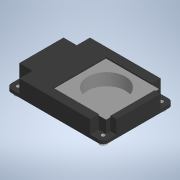
# Autodesk Inventor part: PRI_cooler
Saved by Autodesk Inventor 2022 (Build 260153000, 153)
## iProperties
Created: 2025-03-29
Part Number: PRI_cooler
Material: Типовые
Document SubType Name: Modeling
Designer: akap
Density: 1 g/cm^3
Appearance: По умолчанию
Author: akap
Autodesk Inventor part; units mm, degrees
ref_plane "YZ Plane" through (0, 0, 0) normal (1, 0, 0) x (0, 1, 0)
ref_plane "XZ Plane" through (0, 0, 0) normal (0, 1, 0) x (-1, 0, 0)
ref_plane "XY Plane" through (0, 0, 0) normal (0, 0, 1) x (1, 0, 0)
sketch "Эскиз1" plane through (0, 0, 0) normal (0, 1, 0) x (-1, 0, 0)
  line L0 (-24.5, 20) -> (24.5, 20)
  line L1 (27.5, 17) -> (27.5, -17)
  line L2 (24.5, -20) -> (-24.5, -20)
  line L3 (-27.5, -17) -> (-27.5, 17)
  line L4 (-27.5, 20) -> (27.5, -20) construction
  line L5 (27.5, 20) -> (-27.5, -20) construction
  arc A0 (24.5, -20) -> (27.5, -17) centre (24.5, -17) ccw
  arc A1 (-27.5, -17) -> (-24.5, -20) centre (-24.5, -17) ccw
  arc A2 (-24.5, 20) -> (-27.5, 17) centre (-24.5, 17) ccw
  arc A3 (27.5, 17) -> (24.5, 20) centre (24.5, 17) ccw
  line L6 (-24, 16.5) -> (24, 16.5)
  line L7 (24, 16.5) -> (24, -16.5)
  line L8 (24, -16.5) -> (-24, -16.5)
  line L9 (-24, -16.5) -> (-24, 16.5)
  line L10 (-24, 16.5) -> (24, -16.5) construction
  line L11 (24, 16.5) -> (-24, -16.5) construction
  circle A4 centre (24, 16.5) radius 1
  circle A5 centre (24, -16.5) radius 1
  circle A6 centre (-24, -16.5) radius 1
  circle A7 centre (-24, 16.5) radius 1
  point P0 (0, 0)
  dimension "d0" = 55
  dimension "d1" = 40
  dimension "d2" = 3
  dimension "d3" = 3
  dimension "d30" = 48
  dimension "d31" = 33
  dimension "d32" = 2
  dimension "d33" = 2
  dimension "d34" = 2
  dimension "d35" = 2
  constraints: 24 end point, 8 centre point, 8 point on circle, 8 point on line, 8 tangent, 4 coincident, 4 midpoint, 4 parallel, 2 equal radius, 2 horizontal, 2 perpendicular
  measures "d0" distance of L4.end L5.end
  measures "d1" distance of L5.start L4.end
  measures "d2" radius of A0
  measures "d3" radius of A3
  measures "d30" distance of L7.end L8.end
  measures "d31" distance of L6.end L7.end
  measures "d32" diameter of A4
  measures "d33" diameter of A5
  measures "d34" diameter of A6
  measures "d35" diameter of A7
extrude "Выдавливание1" add sketch "Эскиз1" along normal blind 1.8 contours L0 A3 L1 A0 L2 A1 L3 A2 | L6 A4 L7 A5 L8 A6 L9 A7
sketch "Эскиз2" plane through (0, 1.8, 0) normal (0, 1, 0) x (1, 0, 0)
  line L0 (-5.9, 15) -> (24.1, 15)
  line L1 (24.1, 15) -> (24.1, -15)
  line L2 (24.1, -15) -> (-5.9, -15)
  line L3 (-5.9, -15) -> (-5.9, 15)
  line L4 (-5.9, 15) -> (24.1, -15) construction
  line L5 (24.1, 15) -> (-5.9, -15) construction
  line L6 (27.5, -17) -> (27.5, 17) projected
  line L7 (-27.5, 17) -> (-27.5, -17) projected
  line L8 (-27.5, 0) -> (27.5, 0)
  circle A0 centre (8.45, 0.95) radius 10.65
  line L9 (8.45, 15) -> (8.45, 0.95)
  line L10 (8.45, 11.6) -> (8.45, 15)
  line L11 (-5.9, 0.95) -> (8.45, 0.95)
  line L12 (-5.9, 0.95) -> (-2.2, 0.95)
  point P0 (0, 0)
  point P1 (9.1, 0)
  dimension "d10" = 30
  dimension "d11" = 30
  dimension "d12" = 3.4
  dimension "d13" = 21.3
  dimension "d14" = 3.4
  dimension "d15" = 3.7
  constraints: 22 end point, 7 point on line, 4 midpoint, 2 horizontal, 2 parallel, 2 perpendicular, 2 point on circle, 1 centre point
  measures "d10" distance of L1.end L2.end
  measures "d11" distance of L0.end L1.end
  measures "d12" distance between parallel lines of L6 L1
  measures "d13" diameter of A0
  measures "d14" distance of L10.start L10.end
  measures "d15" distance of L11.start L12.end
extrude "Выдавливание2" add sketch "Эскиз2" along normal blind 6.9 contours L0 L9 A0 L11 L3 | L0 L1 L8 A0 L9 | L11 A0 L8 L3 | L8 A0 L1 L2 L3
sketch "Эскиз3" plane through (0, 1.8, 0) normal (0, 1, 0) x (1, 0, 0)
  line L0 (24.5, 20) -> (-24.5, 20) projected
  arc A0 (-24.5, 20) -> (-27.5, 17) centre (-24.5, 17) ccw projected
  line L1 (-27.5, 17) -> (-27.5, -17) projected
  arc A1 (-27.5, -17) -> (-24.5, -20) centre (-24.5, -17) ccw projected
  line L2 (-24.5, -20) -> (24.5, -20) projected
  arc A2 (24.5, -20) -> (27.5, -17) centre (24.5, -17) ccw projected
  line L3 (27.5, -17) -> (27.5, 17) projected
  arc A3 (27.5, 17) -> (24.5, 20) centre (24.5, 17) ccw projected
  line L4 (-5.9, 15) -> (24.1, 15) projected
  line L5 (24.1, 15) -> (24.1, -15) projected
  line L6 (24.1, -15) -> (-5.9, -15) projected
  line L7 (-5.9, -15) -> (-5.9, 15) projected
  line L8 (24.5, 20) -> (-24.5, 20) projected
  line L9 (-20, 20) -> (-20, -20)
  line L10 (-27.5, 17) -> (-27.5, -17) projected
  line L11 (-27.5, -12.5) -> (27.5, -12.5)
  line L12 (27.5, -17) -> (27.5, 17) projected
  line L13 (20, 20) -> (20, -20)
  line L14 (-24.5, -20) -> (24.5, -20) projected
  line L15 (27.5, 12.5) -> (-27.5, 12.5)
  point P0 (0, 0)
  point P1 (24.1, 12.5)
  point P2 (24.1, -12.5)
  point P3 (-20, 12.5)
  point P4 (-20, -12.5)
  point P5 (20, -15)
  point P6 (20, 15)
  dimension "d18" = 7.5
  dimension "d19" = 7.5
  dimension "d20" = 7.5
  dimension "d21" = 7.5
  constraints: 8 end point, 8 point on line, 4 perpendicular
  measures "d18" distance between parallel lines of L2 L11
  measures "d19" distance between parallel lines of L8 L15
  measures "d20" distance between parallel lines of L10 L9
  measures "d21" distance between parallel lines of L13 L3
extrude "Выдавливание3" add sketch "Эскиз3" along normal blind 7.6 contours L13 L4 L7 L15 L9 L0 | L3 L11 L5 L15 | L15 L7 L11 L9 | L9 L11 L1 L15 | L11 L7 L6 L13 L2 L9
sketch "Эскиз4" plane through (0, 0, 0) normal (0, -1, 0) x (1, 0, 0)
  circle A0 centre (-24, 16.5) radius 1 projected
  circle A1 centre (-24, 16.5) radius 2
  circle A2 centre (-24, -16.5) radius 1 projected
  circle A3 centre (-24, -16.5) radius 2
  circle A4 centre (24, -16.5) radius 1 projected
  circle A5 centre (24, -16.5) radius 2
  circle A6 centre (24, 16.5) radius 1 projected
  circle A7 centre (24, 16.5) radius 2
  point P0 (-24.5, 17)
  point P1 (24.5, 17)
  point P2 (24.5, -17)
  point P3 (-24.5, -17)
  dimension "d36" = 4
  dimension "d37" = 4
  dimension "d38" = 4
  dimension "d39" = 4
  constraints: 4 centre point, 4 coincident
  measures "d36" diameter of A1
  measures "d37" diameter of A3
  measures "d38" diameter of A5
  measures "d39" diameter of A7
extrude "Выдавливание4" add sketch "Эскиз4" along normal blind 2
equation "\"d19\" = d18"
equation "\"d20\" = d18"
equation "\"d21\" = d18"
